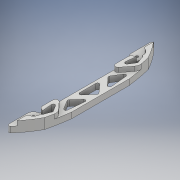
# Autodesk Inventor part: ガイド横上
Saved by Autodesk Inventor 2018.3 (Build 223284000, 284)
## iProperties
Created: 2019-04-06
Part Number: ガイド横上
Material: 一般
Document SubType Name: Modeling
Designer: shun2
Density: 1 g/cm^3
Appearance: 既定
Author: shun2
Autodesk Inventor part; units mm, degrees
ref_plane "YZ Plane" through (0, 0, 0) normal (1, 0, 0) x (0, 1, 0)
ref_plane "XZ Plane" through (0, 0, 0) normal (0, 1, 0) x (-1, 0, 0)
ref_plane "XY Plane" through (0, 0, 0) normal (0, 0, 1) x (1, 0, 0)
sketch "スケッチ1" plane through (0, 0, 0) normal (0, 0, 1) x (1, 0, 0)
  arc A0 (0, 5.1191) -> (3.497, 3.7928) centre (2, 5.1191) ccw
  arc A1 (3.497, 3.7928) -> (20.2574, 27.638) centre (-93.8083, 90) ccw
  arc A2 (20.2574, 27.638) -> (25.3494, 55.5364) centre (-242.442, 90) ccw
  line L0 (25.3494, 55.5364) -> (25.3494, 124.4636)
  arc A3 (25.3494, 124.4636) -> (20.2574, 152.362) centre (-242.442, 90) ccw
  arc A4 (20.2574, 152.362) -> (3.497, 176.2072) centre (-93.8083, 90) ccw
  arc A5 (3.497, 176.2072) -> (0, 174.8809) centre (2, 174.8809) ccw
  line L1 (0, 174.8809) -> (0, 152.362)
  arc A6 (0, 152.362) -> (7, 145.362) centre (7, 152.362) ccw
  line L2 (7, 145.362) -> (7, 109.815)
  line L3 (7, 80.815) -> (7, 34.638)
  arc A7 (7, 34.638) -> (0, 27.638) centre (7, 27.638) ccw
  line L4 (0, 27.638) -> (0, 5.1191)
  arc A8 (20.8277, 125.2984) -> (17.1291, 126.1497) centre (18.8368, 125.1086) ccw
  line L5 (20.8277, 125.2984) -> (22.6836, 105.8325)
  arc A9 (19.2111, 104.2992) -> (22.6836, 105.8325) centre (20.6926, 105.6427) ccw
  line L6 (19.2111, 104.2992) -> (11.0046, 113.3481)
  arc A10 (10.7784, 115.7327) -> (11.0046, 113.3481) centre (12.4861, 114.6917) ccw
  line L7 (10.7784, 115.7327) -> (17.1291, 126.1497)
  arc A11 (18.8075, 140.2289) -> (18.979, 141.9846) centre (17.1068, 141.2812) ccw
  line L8 (18.8075, 140.2289) -> (14.4979, 133.2642)
  arc A12 (10.8061, 134.5052) -> (14.4979, 133.2642) centre (12.7972, 134.3166) ccw
  line L9 (10.8061, 134.5052) -> (12.2009, 149.2292)
  arc A13 (16.0642, 149.7439) -> (12.2009, 149.2292) centre (14.192, 149.0405) ccw
  line L10 (16.0642, 149.7439) -> (18.979, 141.9846)
  arc A14 (14.4979, 46.7358) -> (10.8061, 45.4948) centre (12.7972, 45.6834) ccw
  line L11 (14.4979, 46.7358) -> (18.8075, 39.7711)
  arc A15 (18.979, 38.0154) -> (18.8075, 39.7711) centre (17.1068, 38.7188) ccw
  line L12 (18.979, 38.0154) -> (16.0642, 30.2561)
  arc A16 (12.2009, 30.7708) -> (16.0642, 30.2561) centre (14.192, 30.9595) ccw
  line L13 (12.2009, 30.7708) -> (10.8061, 45.4948)
  arc A17 (11.0046, 66.6519) -> (10.7784, 64.2673) centre (12.4861, 65.3083) ccw
  line L14 (11.0046, 66.6519) -> (19.2111, 75.7008)
  arc A18 (22.6836, 74.1675) -> (19.2111, 75.7008) centre (20.6926, 74.3573) ccw
  line L15 (22.6836, 74.1675) -> (20.8277, 54.7016)
  arc A19 (17.1291, 53.8503) -> (20.8277, 54.7016) centre (18.8368, 54.8914) ccw
  line L16 (17.1291, 53.8503) -> (10.7784, 64.2673)
  arc A20 (13.4987, 101.0407) -> (10, 99.7163) centre (12, 99.7163) ccw
  line L17 (13.4987, 101.0407) -> (22.0846, 91.3243)
  arc A21 (22.0846, 88.6757) -> (22.0846, 91.3243) centre (20.5859, 90) ccw
  line L18 (22.0846, 88.6757) -> (13.4987, 78.9593)
  arc A22 (10, 80.2837) -> (13.4987, 78.9593) centre (12, 80.2837) ccw
  line L19 (10, 80.2837) -> (10, 99.7163)
  circle A23 centre (7, 152.362) radius 1.5
  circle A24 centre (7, 27.638) radius 1.5
  line L20 (7, 109.815) -> (7, 80.815)
  point P0 (0, 0)
  point P1 (0, 0)
  constraints: 46 point on circle, 42 end point, 25 centre point, 1 vertical
extrude "押し出し1" add sketch "スケッチ1" along normal blind 7
sketch "スケッチ2" plane through (0, 0, 7) normal (0, 0, 1) x (1, 0, 0)
  line L0 (7, 52.6381) -> (7, 57.6381)
  line L1 (7, 52.6381) -> (7, 42.6381)
  line L2 (7, 12.6381) -> (7, 8.9003)
  line L3 (7, 42.6381) -> (7, 38.42)
  line L4 (7, 12.6381) -> (7, 16.8562)
  line L5 (7, 141.5801) -> (7, 122.6381)
  line L6 (7, 171.0997) -> (7, 163.1439)
  circle A0 centre (7, 152.362) radius 1.5 projected
  arc A1 (10, 80.2837) -> (13.4987, 78.9593) centre (12, 80.2837) ccw projected
  line L7 (10, 80.2837) -> (10, 99.7163) projected
  arc A2 (13.4987, 101.0407) -> (10, 99.7163) centre (12, 99.7163) ccw projected
  line L8 (13.4987, 101.0407) -> (22.0846, 91.3243) projected
  arc A3 (22.0846, 88.6757) -> (22.0846, 91.3243) centre (20.5859, 90) ccw projected
  line L9 (22.0846, 88.6757) -> (13.4987, 78.9593) projected
  arc A4 (19.2111, 104.2992) -> (22.6836, 105.8325) centre (20.6926, 105.6427) ccw projected
  line L10 (19.2111, 104.2992) -> (11.0046, 113.3481) projected
  arc A5 (10.7784, 115.7327) -> (11.0046, 113.3481) centre (12.4861, 114.6917) ccw projected
  line L11 (10.7784, 115.7327) -> (17.1291, 126.1497) projected
  arc A6 (20.8277, 125.2984) -> (17.1291, 126.1497) centre (18.8368, 125.1086) ccw projected
  line L12 (20.8277, 125.2984) -> (22.6836, 105.8325) projected
  line L13 (11.0046, 66.6519) -> (19.2111, 75.7008) projected
  arc A7 (22.6836, 74.1675) -> (19.2111, 75.7008) centre (20.6926, 74.3573) ccw projected
  line L14 (22.6836, 74.1675) -> (20.8277, 54.7016) projected
  arc A8 (17.1291, 53.8503) -> (20.8277, 54.7016) centre (18.8368, 54.8914) ccw projected
  line L15 (17.1291, 53.8503) -> (10.7784, 64.2673) projected
  arc A9 (11.0046, 66.6519) -> (10.7784, 64.2673) centre (12.4861, 65.3083) ccw projected
  line L16 (14.4979, 46.7358) -> (18.8075, 39.7711) projected
  arc A10 (18.979, 38.0154) -> (18.8075, 39.7711) centre (17.1068, 38.7188) ccw projected
  line L17 (18.979, 38.0154) -> (16.0642, 30.2561) projected
  arc A11 (12.2009, 30.7708) -> (16.0642, 30.2561) centre (14.192, 30.9595) ccw projected
  line L18 (12.2009, 30.7708) -> (10.8061, 45.4948) projected
  arc A12 (14.4979, 46.7358) -> (10.8061, 45.4948) centre (12.7972, 45.6834) ccw projected
  arc A13 (16.0642, 149.7439) -> (12.2009, 149.2292) centre (14.192, 149.0405) ccw projected
  line L19 (16.0642, 149.7439) -> (18.979, 141.9846) projected
  arc A14 (18.8075, 140.2289) -> (18.979, 141.9846) centre (17.1068, 141.2812) ccw projected
  line L20 (18.8075, 140.2289) -> (14.4979, 133.2642) projected
  arc A15 (10.8061, 134.5052) -> (14.4979, 133.2642) centre (12.7972, 134.3166) ccw projected
  line L21 (10.8061, 134.5052) -> (12.2009, 149.2292) projected
  circle A16 centre (7, 27.638) radius 1.5 projected
  circle A17 centre (7, 152.362) radius 1.5 projected
  arc A18 (25.3494, 124.4636) -> (20.2574, 152.362) centre (-242.442, 90) ccw projected
  arc A19 (20.2574, 152.362) -> (3.497, 176.2072) centre (-93.8083, 90) ccw projected
  arc A20 (3.497, 176.2072) -> (0, 174.8809) centre (2, 174.8809) ccw projected
  line L22 (0, 174.8809) -> (0, 152.362) projected
  arc A21 (0, 152.362) -> (7, 145.362) centre (7, 152.362) ccw projected
  line L23 (7, 145.362) -> (7, 34.638) projected
  arc A22 (7, 34.638) -> (0, 27.638) centre (7, 27.638) ccw projected
  line L24 (0, 27.638) -> (0, 5.1191) projected
  arc A23 (0, 5.1191) -> (3.497, 3.7928) centre (2, 5.1191) ccw projected
  arc A24 (3.497, 3.7928) -> (20.2574, 27.638) centre (-93.8083, 90) ccw projected
  arc A25 (20.2574, 27.638) -> (25.3494, 55.5364) centre (-242.442, 90) ccw projected
  line L25 (25.3494, 55.5364) -> (25.3494, 124.4636) projected
  line L26 (7, 171.0997) -> (7, 172.0834)
  arc A26 (20.2574, 152.362) -> (3.497, 176.2072) centre (-93.8083, 90) ccw projected
  line L27 (7, 8.9003) -> (7, 7.9166)
  arc A27 (3.497, 3.7928) -> (20.2574, 27.638) centre (-93.8083, 90) ccw projected
  arc A28 (7, 163.1439) -> (9.6087, 159.3937) centre (11, 163.1439) ccw
  arc A29 (9.6087, 145.3303) -> (7, 141.5801) centre (11, 141.5801) ccw
  arc A30 (9.6087, 20.6064) -> (7, 16.8562) centre (11, 16.8562) ccw
  arc A31 (7, 38.42) -> (9.6087, 34.6698) centre (11, 38.42) ccw
  line L28 (16.0642, 149.7439) -> (18.979, 141.9846) projected
  arc A32 (10, 80.2837) -> (13.4987, 78.9593) centre (12, 80.2837) ccw projected
  line L29 (10, 80.2837) -> (10, 99.7163) projected
  arc A33 (13.4987, 101.0407) -> (10, 99.7163) centre (12, 99.7163) ccw projected
  line L30 (13.4987, 101.0407) -> (22.0846, 91.3243) projected
  arc A34 (22.0846, 88.6757) -> (22.0846, 91.3243) centre (20.5859, 90) ccw projected
  line L31 (22.0846, 88.6757) -> (13.4987, 78.9593) projected
  arc A35 (19.2111, 104.2992) -> (22.6836, 105.8325) centre (20.6926, 105.6427) ccw projected
  line L32 (19.2111, 104.2992) -> (11.0046, 113.3481) projected
  arc A36 (10.7784, 115.7327) -> (11.0046, 113.3481) centre (12.4861, 114.6917) ccw projected
  line L33 (10.7784, 115.7327) -> (17.1291, 126.1497) projected
  arc A37 (20.8277, 125.2984) -> (17.1291, 126.1497) centre (18.8368, 125.1086) ccw projected
  line L34 (20.8277, 125.2984) -> (22.6836, 105.8325) projected
  line L35 (11.0046, 66.6519) -> (19.2111, 75.7008) projected
  arc A38 (22.6836, 74.1675) -> (19.2111, 75.7008) centre (20.6926, 74.3573) ccw projected
  line L36 (22.6836, 74.1675) -> (20.8277, 54.7016) projected
  arc A39 (17.1291, 53.8503) -> (20.8277, 54.7016) centre (18.8368, 54.8914) ccw projected
  line L37 (17.1291, 53.8503) -> (10.7784, 64.2673) projected
  arc A40 (11.0046, 66.6519) -> (10.7784, 64.2673) centre (12.4861, 65.3083) ccw projected
  line L38 (14.4979, 46.7358) -> (18.8075, 39.7711) projected
  arc A41 (18.979, 38.0154) -> (18.8075, 39.7711) centre (17.1068, 38.7188) ccw projected
  line L39 (18.979, 38.0154) -> (16.0642, 30.2561) projected
  arc A42 (12.2009, 30.7708) -> (16.0642, 30.2561) centre (14.192, 30.9595) ccw projected
  line L40 (12.2009, 30.7708) -> (10.8061, 45.4948) projected
  arc A43 (14.4979, 46.7358) -> (10.8061, 45.4948) centre (12.7972, 45.6834) ccw projected
  arc A44 (16.0642, 149.7439) -> (12.2009, 149.2292) centre (14.192, 149.0405) ccw projected
  line L41 (16.0642, 149.7439) -> (18.979, 141.9846) projected
  arc A45 (18.8075, 140.2289) -> (18.979, 141.9846) centre (17.1068, 141.2812) ccw projected
  line L42 (18.8075, 140.2289) -> (14.4979, 133.2642) projected
  arc A46 (10.8061, 134.5052) -> (14.4979, 133.2642) centre (12.7972, 134.3166) ccw projected
  line L43 (10.8061, 134.5052) -> (12.2009, 149.2292) projected
  circle A47 centre (7, 27.638) radius 1.5 projected
  circle A48 centre (7, 152.362) radius 1.5 projected
  arc A49 (25.3494, 124.4636) -> (20.2574, 152.362) centre (-242.442, 90) ccw projected
  arc A50 (20.2574, 152.362) -> (3.497, 176.2072) centre (-93.8083, 90) ccw projected
  arc A51 (3.497, 176.2072) -> (0, 174.8809) centre (2, 174.8809) ccw projected
  line L44 (0, 174.8809) -> (0, 152.362) projected
  arc A52 (0, 152.362) -> (7, 145.362) centre (7, 152.362) ccw projected
  line L45 (7, 145.362) -> (7, 34.638) projected
  arc A53 (7, 34.638) -> (0, 27.638) centre (7, 27.638) ccw projected
  line L46 (0, 27.638) -> (0, 5.1191) projected
  arc A54 (0, 5.1191) -> (3.497, 3.7928) centre (2, 5.1191) ccw projected
  arc A55 (3.497, 3.7928) -> (20.2574, 27.638) centre (-93.8083, 90) ccw projected
  arc A56 (20.2574, 27.638) -> (25.3494, 55.5364) centre (-242.442, 90) ccw projected
  line L47 (25.3494, 55.5364) -> (25.3494, 124.4636) projected
  arc A57 (10.8061, 134.5052) -> (14.4979, 133.2642) centre (12.7972, 134.3166) ccw
  arc A58 (10.8061, 134.5052) -> (14.4979, 133.2642) centre (12.7972, 134.3166) ccw projected
  line L48 (10.8061, 134.5052) -> (11.9652, 146.7409)
  line L49 (14.4979, 133.2642) -> (18.8075, 140.2289)
  line L50 (18.979, 141.9846) -> (16.0642, 149.7439)
  arc A59 (18.8075, 140.2289) -> (18.979, 141.9846) centre (17.1068, 141.2812) ccw
  arc A60 (9.6087, 145.3303) -> (11.9652, 146.7409) centre (7, 152.362) ccw
  arc A61 (14.3811, 151.0316) -> (9.6087, 159.3937) centre (7, 152.362) ccw
  arc A62 (16.0642, 149.7439) -> (14.3811, 151.0316) centre (14.192, 149.0405) ccw
  arc A63 (14.3811, 28.9684) -> (16.0642, 30.2561) centre (14.192, 30.9595) ccw
  arc A64 (14.4979, 46.7358) -> (10.8061, 45.4948) centre (12.7972, 45.6834) ccw
  arc A65 (18.979, 38.0154) -> (18.8075, 39.7711) centre (17.1068, 38.7188) ccw
  line L51 (10.8061, 45.4948) -> (11.9651, 33.2592)
  arc A66 (18.979, 38.0154) -> (18.8075, 39.7711) centre (17.1068, 38.7188) ccw projected
  line L52 (16.0642, 30.2561) -> (18.979, 38.0154)
  line L53 (14.4979, 46.7358) -> (18.8075, 39.7711) projected
  line L54 (18.8075, 39.7711) -> (14.4979, 46.7358)
  arc A67 (9.6087, 20.6064) -> (14.3811, 28.9684) centre (7, 27.6381) ccw
  arc A68 (11.9651, 33.2592) -> (9.6087, 34.6698) centre (7, 27.6381) ccw
  arc A69 (25.3494, 124.4636) -> (20.2574, 152.362) centre (-242.442, 90) ccw projected
  line L55 (23.1699, 138.4797) -> (7, 117.6381)
  line L56 (23.1699, 41.5203) -> (7, 58.8532)
  line L57 (7, 34.638) -> (7, 145.362) projected
  line L58 (7, 57.6381) -> (7, 58.8532)
  line L59 (7, 117.6381) -> (7, 122.6381)
  point P0 (0, 0)
  point P1 (7, 35.1381)
  point P2 (7, 20.1381)
  point P3 (7, 144.862)
  point P4 (7, 159.862)
  dimension "d6" = 4
  constraints: 42 end point, 33 point on circle, 14 centre point, 12 tangent, 9 point on line, 6 coincident, 5 collinear, 4 equal radius, 4 vertical, 2 other
  measures "d6" radius of A28
extrude "押し出し2" add sketch "スケッチ2" along normal blind 5.5 contours L0 L23 L56 A25 A24 L27 L2 L4 A30 A67 A11 L17 A10 L16 A12 L18 A68 A31 L3 L1 | L23 L5 A29 A60 L21 A15 L20 A14 L19 A13 A61 A28 L6 L26 A19 A18 L55
fillet "フィレット1" radius 8 2 edges at (23.1699, 138.4797, 9.75) (23.1699, 41.5203, 9.75)
fillet "フィレット1" radius 3 2 edges at (7, 117.6381, 9.75) (7, 58.8532, 9.75)
